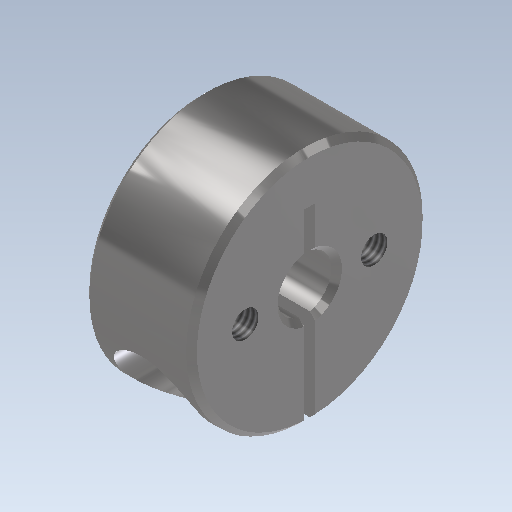
# Autodesk Inventor part: SCS5-10b
Saved by Autodesk Inventor 2021 (Build 250183000, 183)
## iProperties
Created: 2019-11-13
Part Number: SCS5-10b
Material: 鋼、炭素鋼
Catalog Web Link: www.cadenas.de
Description: SCS, PSCS, SSCS, SCSA, SCSAW, SCSAB-b-Set Collars - Slit - Standard Type
Vendor: MISUMI
Document SubType Name: Modeling
Designer: psadmin
Manufacturer: MISUMI
Mass: 3.13365 g
Surface Area: 18.8987 cm^2
Volume: 3.13365 cm^3
Density: 7.85 g/cm^3
Appearance: 半つや出し
Category: PARTsolutions
Company: MISUMI
PSOL_IDENT_0: {$CADENAS_DATA\23d-libs\misumi\metric\03_set_collars\scs_b.prj},199 {VTYP=3D},{NB=SCS5-10b},{LINA=SC
PSOL_IDENT_1: S5-10b},{NN=SCS, PSCS, SSCS, SCSA, SCSAW, SCSAB-b},{DATE=30.03.2018 01:14:40},{GEOMDATE=02.02.2011 0
PSOL_IDENT_2: 0:00:00},{VERSION=},{LINEID=230},{WBVAR=MAT,ST,BS},{WBNUMERIC=BS}  {NB=SCS5-10b},{LINA=SCS5-10b},{KT=
PSOL_IDENT_3: DUMMY},{PN=SCS5-10},{TYPE=SCS},{MAT=1045},{ST=Black Oxide},{AC=Hexagon Socket Head Set Screws (1 Pc.
PSOL_IDENT_4: )},{D=5},{BS=10},{BALG=8,10},{B0=8,10},{B1=8,10},{B2=8},{D1=22},{M=M4},{THMD=4},{THDMIN=3.242},{ST0='
PSOL_IDENT_5: Black Oxide','Black Oxide','Electroless Nickel Plating','Electroless Nickel Plating'},{DD=4.5},{R=3.
PSOL_IDENT_6: 75},{W=1.0},{X=6.500},{Y=4.0},{Z=6~7},{Z1=6.50},{P1=0},{C=0.5},{L=10},{P=0.0},{MATA=  '1045','S45C(1
PSOL_IDENT_7: 045 Steel)(1.1191_C45E (Ck45))','304','SUS304(304 Stainless Steel)(1.4301_X5CrNi18-10)','2017','A201
PSOL_IDENT_8: 7(2017 Aluminum)(EN AW-2017_AlCu4MgSi)'  }
NN: SCS, PSCS, SSCS, SCSA, SCSAW, SCSAB-b
NT: Set Collars - Slit - Standard Type
NB: SCS5-10b
NBSYN: $PN.b
LINA: SCS5-10b
PN: SCS5-10
MAT: 1045 Carbon Steel
ST: Black Oxide
AC: Hexagon Socket Head Set Screws (1 Pc.)
D: 5
BS: 10
D1: 22
M: M4
DD: 4.5
R: 3.75
W: 1
X: 6.5
Y: 4
Z: 6~7
C: 0.5
P: 0
SUPPLIER: MISUMI
ARTICLENO: SCS5-10b
BOMINFO: SCS5-10b
CREATOR: CADENAS GmbH
Title: SCS5-10b
Author: Cadenas PARTsolutions
Comments: Set Collars - Slit - Standard Type
Autodesk Inventor part; units mm, degrees
sketch "Sketch_1" plane through (0, 0, 0) normal (0, 0, 1) x (1, 0, 0)
  line L0 (5, 0) -> (-5, 0)
  line L1 (-5, 10.5) -> (-5, 3)
  line L2 (-5, 3) -> (-4.5, 2.5)
  line L3 (-4.5, 2.5) -> (4.5, 2.5)
  line L4 (4.5, 2.5) -> (5, 3)
  line L5 (5, 3) -> (5, 10.5)
  line L6 (5, 10.5) -> (4.5, 11)
  line L7 (4.5, 11) -> (-4.5, 11)
  line L8 (-4.5, 11) -> (-5, 10.5)
  constraints: 18 end point
revolve "Revolution1" add sketch "Sketch_1" angle 360 about axis through (5, 0, 0) along (1, 0, 0)
sketch "Sketch_2" plane through (0, 0, 0) normal (1, 0, 0) x (0, 1, 0)
  line L0 (-11, 0.5) -> (-11, -0.5)
  line L1 (-11, -0.5) -> (6.5, -0.5)
  line L2 (6.5, -0.5) -> (6.5, 0.5)
  line L3 (6.5, 0.5) -> (-11, 0.5)
  constraints: 8 end point
extrude "Extrusion1" cut sketch "Sketch_2" along normal mid plane 10
sketch "Sketch_3" plane through (0, 0, 0) normal (1, 0, 0) x (0, 1, 0)
  line L0 (-6.5, 11) -> (-6.5, 0)
  line L1 (-6.5, 0) -> (-8.75, 0)
  line L2 (-8.75, 0) -> (-8.75, 4)
  line L3 (-8.75, 4) -> (-10.25, 4)
  line L4 (-10.25, 4) -> (-10.25, 11)
  line L5 (-10.25, 11) -> (-6.5, 11)
  line L6 (-6.5, 11) -> (-6.5, 0)
  constraints: 14 end point
revolve "Revolution2" cut sketch "Sketch_3" angle 360 about axis through (0, -6.5, 11) along (0, 0, 1)
sketch "Sketch4" plane through (-4.5, -2.4495, -0.5) normal (0, 0, 1) x (1, 0, 0)
  point P0 (4.5, -4.0505)
hole "Hole1" at (0, -6.5, -0.5) direction (0, 0, -1) diameter 3.242 depth 9.75 countersink diameter 4 countersink angle 90 thread size "M4x0.7" class "6H" standard "ISO Metric profile"
ref_plane "body_screw_XY" through (0, -6.5, 4) normal (0, 0, 1) x (1, 0, 0)
ref_plane "body_screw_YZ" through (0, -6.5, 4) normal (1, 0, 0) x (0, 1, 0)
ref_plane "body_screw_ZX" through (0, -6.5, 4) normal (0, 1, 0) x (0, 0, 1)
sketch "スケッチ5" plane through (5, 0, 0) normal (1, 0, 0) x (0, 0, -1)
  line L0 (0, 0) -> (-6, 0)
  point P0 (6, 0)
  dimension "d12" = 6
  dimension "d15" = 360
  constraints: 2 end point, 1 coincident, 1 horizontal, 3 other
  measures "d12" distance of L0.start L0.end
hole "穴2" at (5, 0, 6) at (5, 0, -6) direction (-1, 0, 0) diameter 2.459 depth 8.8 thread size "M3x0.5" class "6H" standard "ISO Metric profile"
body "Solid1"
